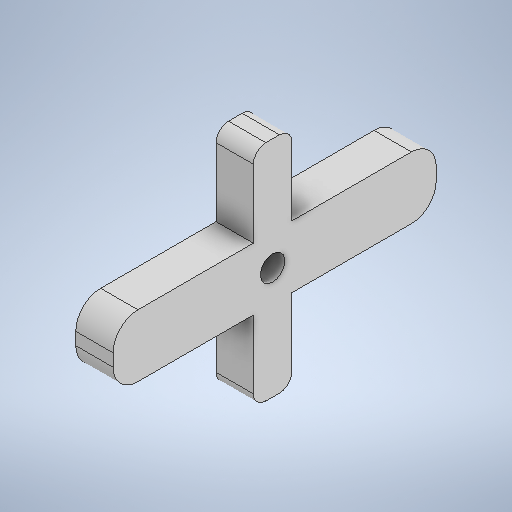
# Autodesk Inventor part: 6P-016 cutout
Saved by Autodesk Inventor 2025.2 (Build 292293000, 293)
## iProperties
Created: 2025-02-17
Part Number: 6P-016 cutout
Material: Generic
Document SubType Name: Modeling
Designer: lachl
Density: 1 g/cm^3
Appearance: Default
Category: <PART CATAGORY>
Title: <TITLE>
Author: lachl
Revision Number: 1
Autodesk Inventor part; units mm, degrees
ref_plane "YZ Plane" through (0, 0, 0) normal (1, 0, 0) x (0, 1, 0)
ref_plane "XZ Plane" through (0, 0, 0) normal (0, 1, 0) x (-1, 0, 0)
ref_plane "XY Plane" through (0, 0, 0) normal (0, 0, 1) x (1, 0, 0)
sketch "Sketch6" plane through (0, 0, 0) normal (1, 0, 0) x (0, 1, 0)
  point P0 (0, 0)
sketch "Sketch7" plane through (0, 0, 0) normal (1, 0, 0) x (0, 1, 0)
  line L0 (-2.5, -13.1614) -> (2.5, -13.1614)
  line L1 (2.5, 12.8386) -> (-2.5, 12.8386)
  circle A0 centre (0, 0) radius 0.9858
  line L2 (9, 1.55) -> (9, -1.55)
  line L3 (-9, -1.55) -> (-9, 1.55)
  line L4 (2.5, 1.55) -> (9, 1.55)
  line L5 (-9, 1.55) -> (-2.5, 1.55)
  line L6 (-2.5, -1.55) -> (-9, -1.55)
  line L7 (9, -1.55) -> (2.5, -1.55)
  line L8 (2.5, 1.55) -> (2.5, 12.8386)
  line L9 (2.5, -13.1614) -> (2.5, -1.55)
  line L10 (-2.5, -1.55) -> (-2.5, -13.1614)
  line L11 (-2.5, 12.8386) -> (-2.5, 1.55)
  point P0 (-9, 0)
  point P1 (0, 12.8386)
  point P2 (9, 0)
  point P3 (0, -13.1614)
  dimension "d85" = 5
  dimension "d86" = 3.1
  dimension "d90" = 26
  dimension "d91" = 3.1
  dimension "d92" = 5
  dimension "d93" = 18
  constraints: 24 end point, 10 parallel, 4 midpoint, 4 perpendicular, 3 coincident, 3 horizontal, 2 horizontal alignment, 2 vertical alignment, 1 centre point
  measures "d85" distance of L11.start L8.end
  measures "d86" distance between parallel lines of L6 L5
  measures "d90" distance from line of L0 point (0, 12.839)
  measures "d91" distance of L2.start L2.end
  measures "d92" distance of L0.start L9.start
  measures "d93" distance between parallel lines of L3 L2
extrude "Extrusion3" add sketch "Sketch7" along normal blind 3
fillet "Fillet1" radius 1 1 edges at (1.5, 9, 1.55)
fillet "Fillet2" radius 1 1 edges at (1.5, 9, -1.55)
fillet "Fillet3" radius 1 1 edges at (1.5, -9, -1.55)
fillet "Fillet4" radius 1 1 edges at (1.5, -9, 1.55)
fillet "Fillet5" radius 2 1 edges at (1.5, -2.5, 12.8386)
fillet "Fillet6" radius 2 1 edges at (1.5, 2.5, 12.8386)
fillet "Fillet7" radius 2 1 edges at (1.5, 2.5, -13.1614)
fillet "Fillet8" radius 2 1 edges at (1.5, -2.5, -13.1614)
body "Solid2"
